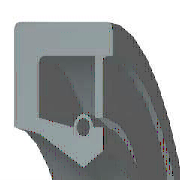
# Autodesk Inventor part: IS0 6194/1 - 25x52x7-Type 3
Saved by Autodesk Inventor 2023.2 (Build 272271030, 271C)
## iProperties
Created: 2022-02-04
Part Number: IS0 6194/1 - 25x52x7-Type 3
Material: Rubber
Description: Rotary shaft lip type seals 3 - Assembled
Document SubType Name: Modeling
Standard: ISO 6194/1
Designer: admin
Standards Organization: ISO
Language: en-US
Size Designation: 25x52x7-Type 3
Categories: <MemberInstance><Categories><Category DisplayName="Shaft Parts" InternalName="7f7aeb1f-a693-4053-b835-cee3144e0d98" Mnemonic="SHFT"><Category DisplayName="Sealing" InternalName="7cc80d44-b28a-4eb5-95d8-e54d452fb95e" Mnemonic="GSKT"><Category DisplayName="Lip Seals" InternalName="b1bc488c-c02d-4af6-ad2b-51fbaea8c3f6" Mnemonic="SLGSKT"><CategoryParameter DisplayName="Shaft Diameter" InternalName="0ca11fbe-a678-4712-b689-66c4985a82dc" Mnemonic="shaftdia"/><CategoryParameter DisplayName="Outer Diameter" InternalName="71be0bee-fd03-42a6-9991-d2da44fa6dc2" Mnemonic="outdia"/><CategoryParameter DisplayName="Thickness" InternalName="c704564b-74bd-4c14-a078-fb73c2ed3f11" Mnemonic="thick"/><CategoryParameter DisplayName="Size Designation" InternalName="db3ff616-f16a-4b30-8ba9-6c8f0071faba" Mnemonic="sizedes"/></Category></Category></Category><Category DisplayName="DataType" InternalName="23b78d0f-2648-40c6-8793-ca6db495c9e8" Mnemonic="DATATYPE"><CategoryParameter DisplayName="DisplayName" InternalName="05415f3d-3907-474b-a020-eb9d644f4cf3" Mnemonic="DISPLAYNAME"/><CategoryParameter DisplayName="Standard" InternalName="0c0a119c-1e12-4c84-803f-101930972f5e" Mnemonic="STANDARD"/><CategoryParameter DisplayName="Description" InternalName="13903e3d-64b1-4950-80da-f627842ea37f" Mnemonic="DESCRIPTION"/><CategoryParameter DisplayName="Designation" InternalName="2675968c-4ce5-49e0-a4f5-552d29089031" Mnemonic="DESIGNATION"/><CategoryParameter DisplayName="Default Row" InternalName="2af9ec52-faaa-4026-b378-f9fa4afca842" Mnemonic="DEFAULTROW"/><CategoryParameter DisplayName="Folder Name" InternalName="3f06958e-8713-4116-9be7-ed6184ecc97b" Mnemonic="FOLDERNAME"/><CategoryParameter DisplayName="Revision Guid" InternalName="45a75005-10b1-4dfc-8d6d-dfe629f0b93c" Mnemonic="REVISIONGUID"/><CategoryParameter DisplayName="FileName" InternalName="8b46a4cc-9585-4fed-90c3-899f57e09a73" Mnemonic="FILENAME"/><CategoryParameter DisplayName="StdsOrg" InternalName="8f5914e1-4693-403f-8ab5-d37768198c9d" Mnemonic="STDSORG"/><CategoryParameter DisplayName="Family Version" InternalName="914462f6-6e19-4b14-ba84-155b9680b1d0" Mnemonic="FAMILYREVISION"/><CategoryParameter DisplayName="Standard Revision" InternalName="91d5a463-65c2-4fde-b823-3b7fea5e8e17" Mnemonic="STANDARDREVISION"/><CategoryParameter DisplayName="Member Revision" InternalName="a65d44b9-392f-4f4f-857b-e4b3d54996fe" Mnemonic="MEMBERREVISION"/><CategoryParameter DisplayName="ClipFormat" InternalName="bc51e27b-3422-4e78-93ef-cec197ddf230" Mnemonic="CLIPFORMAT"/><CategoryParameter DisplayName="Manufacturer" InternalName="cd6c7a72-a28a-4e50-99a9-2c7f4e13e5ad" Mnemonic="MANUFACTURER"/><CategoryParameter DisplayName="InternalName" InternalName="cf1d0246-76d9-4b4a-8305-fa0409afb5c1" Mnemonic="INTERNALNAME"/><CategoryParameter DisplayName="IsMetric" InternalName="e2385c5b-1ea4-4823-96a8-8de651266ec3" Mnemonic="ISMETRIC"/><Category DisplayName="Part" InternalName="c0e0b642-3bcb-4cc8-9e80-f96d35c4afa4" Mnemonic="PART"><CategoryParameter DisplayName="Part Number" InternalName="016b6077-bfbe-49bd-92c9-d8d59c39c941" Mnemonic="PARTNUMBER"/><CategoryParameter DisplayName="Stock Number" InternalName="4dba7c1c-e26c-444e-836c-b08b433409a8" Mnemonic="STOCKNUMBER"/><CategoryParameter DisplayName="Material Key" InternalName="5c9a8adb-dd2b-4535-b97f-0a94a95fe41f" Mnemonic="MATERIALKEY"/><CategoryParameter DisplayName="Material" InternalName="818a152a-d3c3-49ca-80ee-df7d91421b8e" Mnemonic="MATERIAL"/></Category></Category><Category DisplayName="Legacy Map DA" InternalName="924fff40-ddd0-4eff-ad42-30e3774ef79e" Mnemonic="LEGACYMAPDA"><CategoryParameter DisplayName="DACookie" InternalName="316934ee-8fe1-4c7a-9c36-f2d79e1add1a" Mnemonic="DACOOKIE"/></Category></Categories><FamilyTemplate Id="i619413"><FamilyTemplateParameters><FamilyTemplateParameter ObjectType="kUserParameterObject" ValueType="xs:double" Id="1" ObjectReferenceKey="Diam"/><FamilyTemplateParameter ObjectType="kUserParameterObject" ValueType="xs:double" Id="2" ObjectReferenceKey="dd"/><FamilyTemplateParameter ObjectType="kUserParameterObject" ValueType="xs:double" Id="3" ObjectReferenceKey="b"/><FamilyTemplateParameter ObjectType="kPropertyObject" ValueType="xs:string" Id="100" ObjectReferenceKey="{32853F0F-3444-11d1-9E93-0060B03C1CA6}" SubObjectId="52"/><FamilyTemplateParameter ObjectType="kPropertyObject" ValueType="xs:string" Id="105" ObjectReferenceKey="{32853F0F-3444-11d1-9E93-0060B03C1CA6}" SubObjectId="5"/><FamilyTemplateParameter ObjectType="kPartComponentDefinitionObject" ValueType="xs:string" Id="110" SubObjectId="Material"/></FamilyTemplateParameters></FamilyTemplate><CategoryParameterMap><ParamToTemplateMap><ParamToTemplate CategoryParameter="//CategoryParameter[@InternalName='05415f3d-3907-474b-a020-eb9d644f4cf3']" ConstantValue="ISO 6194/1"/><ParamToTemplate CategoryParameter="//CategoryParameter[@InternalName='cf1d0246-76d9-4b4a-8305-fa0409afb5c1']" ConstantValue="63F2DD6F-DB27-4715-99D9-29ED097A2E26"/><ParamToTemplate CategoryParameter="//CategoryParameter[@InternalName='3f06958e-8713-4116-9be7-ed6184ecc97b']" ConstantValue="ISO 6194/1(4)"/><ParamToTemplate CategoryParameter="//CategoryParameter[@InternalName='914462f6-6e19-4b14-ba84-155b9680b1d0']" ConstantValue="10"/><ParamToTemplate CategoryParameter="//CategoryParameter[@InternalName='bc51e27b-3422-4e78-93ef-cec197ddf230']" ConstantValue="CF_INVENTOR.STDPARTS"/><ParamToTemplate CategoryParameter="//CategoryParameter[@InternalName='e2385c5b-1ea4-4823-96a8-8de651266ec3']" ConstantValue="true"/><ParamToTemplate CategoryParameter="//CategoryParameter[@InternalName='13903e3d-64b1-4950-80da-f627842ea37f']" ConstantValue="Rotary shaft lip type seals 3 - Assembled"/><ParamToTemplate CategoryParameter="//CategoryParameter[@InternalName='8f5914e1-4693-403f-8ab5-d37768198c9d']" ConstantValue="ISO"/><ParamToTemplate CategoryParameter="//CategoryParameter[@InternalName='0c0a119c-1e12-4c84-803f-101930972f5e']" ConstantValue="ISO 6194/1"/><ParamToTemplate CategoryParameter="//CategoryParameter[@InternalName='cd6c7a72-a28a-4e50-99a9-2c7f4e13e5ad']" TemplateParameter="104"/><ParamToTemplate CategoryParameter="//CategoryParameter[@InternalName='91d5a463-65c2-4fde-b823-3b7fea5e8e17']" TemplateParameter="103"/><ParamToTemplate CategoryParameter="//CategoryParameter[@InternalName='45a75005-10b1-4dfc-8d6d-dfe629f0b93c']" ConstantValue="ee8d8011-fd96-4ae7-b40e-a273b16274f0"/><ParamToTemplate CategoryParameter="//CategoryParameter[@InternalName='2af9ec52-faaa-4026-b378-f9fa4afca842']" ConstantValue="10"/><ParamToTemplate CategoryParameter="//CategoryParameter[@InternalName='8b46a4cc-9585-4fed-90c3-899f57e09a73']" ConstantValue="ISO 6194/1 - 25x52x7-Type 3"/><ParamToTemplate CategoryParameter="//CategoryParameter[@InternalName='a65d44b9-392f-4f4f-857b-e4b3d54996fe']" ConstantValue="54E0E4D5-2D1D-427A-A6E0-0DBD4C35CC2A"/><ParamToTemplate CategoryParameter="//CategoryParameter[@InternalName='db3ff616-f16a-4b30-8ba9-6c8f0071faba']" ConstantValue="25x52x7"/><ParamToTemplate CategoryParameter="//CategoryParameter[@InternalName='316934ee-8fe1-4c7a-9c36-f2d79e1add1a']" ConstantValue="*ISO~I61941C~25~52~7*"/><ParamToTemplate CategoryParameter="//CategoryParameter[@InternalName='2675968c-4ce5-49e0-a4f5-552d29089031']" TemplateParameter="100"/><ParamToTemplate CategoryParameter="//CategoryParameter[@InternalName='0ca11fbe-a678-4712-b689-66c4985a82dc']" TemplateParameter="1"/><ParamToTemplate CategoryParameter="//CategoryParameter[@InternalName='818a152a-d3c3-49ca-80ee-df7d91421b8e']" TemplateParameter="110"/><ParamToTemplate CategoryParameter="//CategoryParameter[@InternalName='016b6077-bfbe-49bd-92c9-d8d59c39c941']" TemplateParameter="105"/><ParamToTemplate CategoryParameter="//CategoryParameter[@InternalName='c704564b-74bd-4c14-a078-fb73c2ed3f11']" TemplateParameter="3"/></ParamToTemplateMap></CategoryParameterMap></MemberInstance>
Density: 0.93 g/cm^3
Appearance: Rubber - Black - Version 1.1
IsCustomPart: 0
Author: admin
Autodesk Inventor part; units mm, degrees
note: some values were not read from the file. Left out: dimensions or parameters whose unit could not be read.
ref_plane "YZ Plane" through (0, 0, 0) normal (1, 0, 0) x (0, 1, 0)
ref_plane "WorkPlane2" through (0, 0, 0) normal (0, 0, 1) x (1, 0, 0)
sketch "Sketch1" plane through (0, 0, 0) normal (0, 1, 0) x (-1, 0, 0)
  point P0 (0, 0)
ref_plane "WorkPlane3" through (0, 0, -7) normal (0, 0, 1) x (1, 0, 0)
sketch "Sketch2" plane through (0, 0, 0) normal (0, 1, 0) x (-1, 0, 0)
  line L0 (16.55, -0.7) -> (25.3, -0.7)
  line L1 (16.55, -0.35) -> (16.55, -0.7)
  line L2 (23.3, -0.35) -> (16.55, -0.35)
  line L3 (23.3, 0) -> (23.3, -0.35)
  line L4 (26, 0) -> (23.3, 0)
  line L5 (26, -7) -> (26, 0)
  line L6 (15.2, -7) -> (26, -7)
  line L7 (14.525, -4.0833) -> (15.2, -7)
  line L8 (13.85, -3.5) -> (14.525, -4.0833)
  line L9 (12.5, -1.75) -> (13.85, -3.5)
  line L10 (13.85, -1.05) -> (12.5, -1.75)
  line L11 (16.55, -1.05) -> (13.85, -1.05)
  line L12 (16.55, -1.05) -> (16.55, -6.3)
  line L13 (25.3, -6.3) -> (16.55, -6.3)
  line L14 (25.3, -0.7) -> (25.3, -6.3)
  line L15 (0, -15.959) -> (0, -1.7548) construction
  line L16 (0, -15.959) -> (0, -1.7548)
  line L17 (0, -19.1509) -> (0, 3.1918) projected
  line L18 (-5.2, 0) -> (31.2, 0) projected
  dimension "d2" = 7
  dimension "d4" = 0.35
  dimension "d6" = 0.35
  dimension "d8" = 0.35
  dimension "d10" = 0.7
  dimension "d12" = 0.7
  dimension "d14" = 2.7
  dimension "d16" = 2.7
  dimension "d18" = 2.9167
  dimension "d20" = 1.75
  dimension "d22" = 1.35
  dimension "d24" = 0.7
  dimension "d26" = 0.675
  dimension "d28" = 1.35
  dimension "d30" = 0.675
  dimension "msp_d33" = 25
  dimension "msp_d34" = 52
  constraints: 34 end point, 6 horizontal, 6 vertical, 3 collinear
  measures "d2" distance of L5.start L4.start
  measures "d4" distance of L3.start L2.start
  measures "d6" distance of L1.start L0.start
  measures "d8" distance of L11.start L0.start
  measures "d10" horizontal distance of L13.start L5.start
  measures "d12" vertical distance of L12.end L6.start
  measures "d14" distance of L4.start L3.start
  measures "d16" distance of L11.start L10.start
  measures "d18" vertical distance of L7.start L6.start
  measures "d20" vertical distance of L9.start L8.start
  measures "d22" horizontal distance of L10.start L9.start
  measures "d24" vertical distance of L10.start L9.start
  measures "d26" horizontal distance of L7.start L6.start
  measures "d28" horizontal distance of L9.start L8.start
  measures "d30" horizontal distance of L8.start L7.start
  measures "msp_d33" diameter of L9.start L15
  measures "msp_d34" diameter of L5 L15
revolve "Revolution1" add sketch "Sketch2" angle 360 about axis through (0, 0, -15.959) along (0, 0, -1)
fillet "Fillet1" radius 0.35 4 edges at (26, 0, 0) (26, 0, -7) (14.525, 0, -4.0833) (16.55, 0, -1.05)
equation "\"d32\" = 0.05 * b"
equation "\"d2\" = b"
equation "\"d4\" = 0.05 * b"
equation "\"d6\" = 0.05 * b"
equation "\"d8\" = 0.05 * b"
equation "\"d10\" = 0.1 * b"
equation "\"d12\" = 0.1 * b"
equation "\"d14\" = 0.1 * dd - 0.1 * Diam"
equation "\"d16\" = 0.1 * dd - 0.1 * Diam"
equation "\"d18\" = 0.416667 * b"
equation "\"d20\" = 0.25 * b"
equation "\"d22\" = 0.05 * dd - 0.05 * Diam"
equation "\"d24\" = 0.1 * b"
equation "\"d26\" = 0.025 * dd - 0.025 * Diam"
equation "\"d28\" = 0.05 * dd - 0.05 * Diam"
equation "\"d30\" = 0.025 * dd - 0.025 * Diam"
equation "\"msp_d33\" = Diam"
equation "\"msp_d34\" = dd"
equation "\"dd\" = 52"
equation "\"Diam\" = 25"
body "Solid1"
